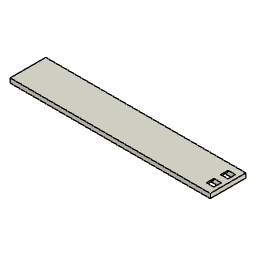
unsorted_smarties_top_panel (Autodesk Fusion 360 design; units mm, degrees)
Autodesk Fusion 360 part; units mm, degrees
sketch "Unsorted Smarties Top" plane through (0, 0, 0) normal (0, 0, 1) x (1, 0, 0)
  line L0 (0, 0) -> (270, 0)
  line L1 (270, 0) -> (270, 48)
  line L2 (270, 48) -> (0, 48)
  line L3 (0, 48) -> (0, 0)
  dimension "d1" = 270
  dimension "d2" = 48
  constraint horizontal L0
  constraint vertical L1
  constraint horizontal L2
  constraint vertical L3
  constraint coincident L0.start L3.end
  measures "d1" distance of L0.start L0.end
  measures "d2" distance of L0.end L1.end
extrude "Extrude1" add sketch "Unsorted Smarties Top" along normal blind 6
sketch "Sketch2" plane through (0, 0, 0) normal (0, 0, -1) x (1, 0, 0)
  line L0 (0, 0) -> (0, -48)
  line L1 (0, -48) -> (270, -48)
  line L2 (270, -48) -> (270, 0)
  line L3 (270, 0) -> (0, 0)
  line L4 (5, -10) -> (265, -10)
  line L5 (265, -10) -> (265, -20)
  line L6 (265, -20) -> (5, -20)
  line L7 (5, -20) -> (5, -10)
  line L8 (5, -29) -> (265, -29)
  line L9 (265, -29) -> (265, -39)
  line L10 (265, -39) -> (5, -39)
  line L11 (5, -39) -> (5, -29)
  dimension "d6" = 5
  dimension "d7" = 5
  dimension "d8" = 5
  dimension "d9" = 5
  dimension "d10" = 10
  dimension "d11" = 10
  dimension "d12" = 9
  dimension "d13" = 10
  constraint horizontal L4
  constraint vertical L5
  constraint horizontal L6
  constraint vertical L7
  constraint horizontal L8
  constraint vertical L9
  constraint horizontal L10
  constraint vertical L11
  measures "d6" distance of L2 L5
  measures "d7" distance of L2 L9
  measures "d8" distance of L0 L7
  measures "d9" distance of L0 L11
  measures "d10" distance of L4.start L6.end
  measures "d11" distance of L3 L4
  measures "d12" distance of L6 L8
  measures "d13" distance of L8.start L10.end
extrude "Extrude2" cut sketch "Sketch2" against normal blind 4 contours L4 L5 L6 L7 | L8 L9 L10 L11
sketch "Sketch3" plane through (0, 0, 4) normal (0, 0, -1) x (1, 0, 0)
  line L0 (5, -20) -> (265, -20)
  line L1 (265, -20) -> (265, -10)
  line L2 (265, -10) -> (5, -10)
  line L3 (5, -10) -> (5, -20)
  line L4 (265, -10) -> (255, -10)
  line L5 (255, -10) -> (255, -20)
  line L6 (255, -20) -> (265, -20)
  line L7 (265, -20) -> (265, -10)
  line L8 (265, -29) -> (255, -29)
  line L9 (255, -29) -> (255, -39)
  line L10 (255, -39) -> (265, -39)
  line L11 (265, -39) -> (265, -29)
  constraint horizontal L4
  constraint vertical L5
  constraint horizontal L6
  constraint vertical L7
  constraint coincident L0 L5.end
  constraint coincident L1.end L2.start
  constraint horizontal L8
  constraint vertical L9
  constraint horizontal L10
  constraint vertical L11
extrude "Extrude3" cut sketch "Sketch3" against normal blind 2 contours L0 L1 L2 L4 L5 L6 L7 | L8 L9 L10 L11
equation "mdfThickness = 6 mm" comment "Thickness of the MDF fibre board"
equation "d4 = mdfThickness"
named bodies: "Unsorted Smarties Top Panel"
